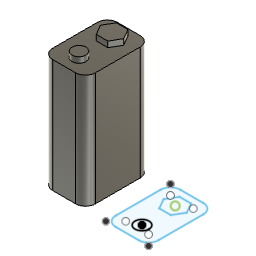
battery (Autodesk Fusion 360 design; units mm, degrees)
Autodesk Fusion 360 part; units mm, degrees
note: some values were not read from the file. Chosen so that the rebuilt part matches the saved one: that a step has no effect.
extrude "Extrude3" [no effect]
extrude "Extrude4" [no effect]
extrude "Extrude5" [no effect]
extrude "Extrude6" [no effect]
extrude "Extrude7" [no effect]
sketch "battery" plane through (0, 0, 0) normal (0, 0, 1) x (1, 0, 0)
  line L0 (29.4, 0) -> (38.6, 0)
  line L1 (42.6, 4) -> (42.6, 22)
  line L2 (38.6, 26) -> (29.4, 26)
  line L3 (25.4, 22) -> (25.4, 4)
  circle A0 centre (34, 5.95) radius 2.8
  line L4 (31.682, 23.3617) -> (29.3235, 19.3234)
  line L5 (29.3235, 19.3234) -> (31.6415, 15.2618)
  line L6 (31.6415, 15.2618) -> (36.318, 15.2383)
  line L7 (36.318, 15.2383) -> (38.6765, 19.2766)
  line L8 (38.6765, 19.2766) -> (36.3585, 23.3382)
  line L9 (36.3585, 23.3382) -> (31.682, 23.3617)
  arc A1 (29.4, 26) -> (25.4, 22) centre (29.4, 22) ccw
  arc A2 (42.6, 22) -> (38.6, 26) centre (38.6, 22) ccw
  arc A3 (38.6, 0) -> (42.6, 4) centre (38.6, 4) ccw
  arc A4 (25.4, 4) -> (29.4, 0) centre (29.4, 4) ccw
  point P0 (25.4, 0)
  point P1 (42.6, 0)
  point P2 (25.4, 26)
  point P3 (34, 19.3)
  point P4 (34, 5.95)
  dimension "d25" = 17.2
  dimension "d26" = 26
  dimension "d27" = 5.6
  dimension "d28" = 4.05
  dimension "d29" = 4
  constraint horizontal L0
  constraint vertical L1
  constraint horizontal L2
  constraint vertical L3
  constraint coincident P4 A0.centre
  constraint coincident P2 L2
  constraint coincident P2 L3
  constraint tangent L2 A1
  constraint tangent L3 A1
  constraint tangent L1 A2
  constraint tangent L2 A2
  constraint equal A1 A2
  constraint coincident P1 L0
  constraint coincident P1 L1
  constraint tangent L0 A3
  constraint tangent L1 A3
  constraint equal A1 A3
  constraint coincident P0 L0
  constraint coincident P0 L3
  constraint tangent L0 A4
  constraint tangent L3 A4
  constraint equal A1 A4
  measures "d25" distance of P0 P1
  measures "d26" distance of P0 P2
  measures "d27" diameter of A0
  measures "d28" distance of P3 L9
  measures "d29" radius of A1
extrude "Extrude8" add sketch "battery" along normal blind 48 contours A0 | L4 L5 L6 L7 L8 L9 makes body 1 at (34.7997, 23.346, 16) makes body 2 at (36.7965, 5.8104, 32)
extrude "Extrude9" add sketch "battery" along normal blind 45.7 bodies 1 2
move_body "Move5" bodies 1 to x (1, 0, 0) y (0, 1, 0) z (0, 0, 1) at (-25.4, 0, 0)
extrude "Extrude10" [suppressed]
extrude "Extrude11" [suppressed]
move_body "Move1" [suppressed]
move_body "Move2" [suppressed]
move_body "Move3" [suppressed]
other "SplitFace1"
split "Split1" [suppressed]
move_body "Move4" [suppressed]
shell "Shell1" [suppressed]
split "Split2" [suppressed]
delete_body "RemoveBody1" bodies 3
split "Split3" [suppressed]
delete_body "RemoveBody2" bodies 4
delete_body "RemoveBody3" bodies 5
named bodies: "battery"
